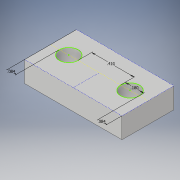
# Autodesk Inventor part: Rectangular Bottom Washer v1.2
Saved by Autodesk Inventor 2019 (Build 230136000, 136)
## iProperties
Created: 2020-01-11
Part Number: Rectangular Bottom Washer v1.2
Material: Generic
Document SubType Name: Modeling
Designer: Obscure_Decision
Density: 1 g/cm^3
Appearance: Default
Author: Obscure_Decision
Autodesk Inventor part; units mm, degrees
ref_plane "YZ Plane" through (0, 0, 0) normal (1, 0, 0) x (0, 1, 0)
ref_plane "XZ Plane" through (0, 0, 0) normal (0, 1, 0) x (-1, 0, 0)
ref_plane "XY Plane" through (0, 0, 0) normal (0, 0, 1) x (1, 0, 0)
sketch "Spacer 2D" plane through (0, 0, 0) normal (0, 1, 0) x (-1, 0, 0)
  line L0 (12.4883, 0) -> (12.4883, -12.7) construction
  line L1 (24.4009, -12.7) -> (0.5757, -12.7)
  line L2 (0.5757, -12.7) -> (0.5757, 0)
  line L3 (0.5757, 0) -> (24.4009, 0)
  line L4 (24.4009, 0) -> (24.4009, -12.7)
  line L5 (24.4009, -12.7) -> (0.5757, 0) construction
  line L6 (0.5757, -12.7) -> (24.4009, 0) construction
  point P0 (0, 0)
  point P1 (12.4883, -6.35)
  dimension "d17" = 23.8252
  dimension "d18" = 12.7
  constraints: 14 end point, 3 midpoint, 2 parallel, 1 horizontal, 1 perpendicular
  measures "d17" distance of L2.end L3.end
  measures "d18" distance of L3.end L1.start
extrude "Spacer Body" add sketch "Spacer 2D" along normal blind 5.08
sketch "Spacer Circles" plane through (0, 5.08, 0) normal (0, 1, 0) x (1, 0, 0)
  line L0 (-0.5757, 0) -> (-0.5757, 12.7) construction
  line L1 (-7.2813, 6.35) -> (-0.5757, 6.35) construction
  line L2 (-7.2813, 6.35) -> (-2.7093, 6.35) construction
  circle A0 centre (-4.9953, 6.35) radius 2.286
  line L3 (-17.6953, 6.35) -> (-7.2813, 6.35) construction
  line L4 (-17.6953, 6.35) -> (-24.4009, 6.35) construction
  line L5 (-24.4009, 12.7) -> (-24.4009, 0) construction
  line L6 (-0.5757, 0) -> (-24.4009, 0) construction
  line L7 (-24.4009, 0) -> (-24.4009, 12.7) construction
  line L8 (-24.4009, 12.7) -> (-0.5757, 12.7) construction
  line L9 (-0.5757, 12.7) -> (-0.5757, 0) construction
  line L10 (-12.4883, 6.35) -> (-12.4883, 0) construction
  line L11 (-24.4009, 0) -> (-0.5757, 0) construction
  circle A1 centre (-19.9813, 6.35) radius 2.286
  dimension "d25" = 4.572
  dimension "d26" = 10.414
  dimension "d31" = 2.1336
  dimension "d32" = 2.1336
  constraints: 18 end point, 5 midpoint, 2 horizontal, 2 parallel, 2 perpendicular, 1 centre point, 1 horizontal alignment, 1 point on line, 1 symmetric about line, 3 other
  measures "d25" distance of L1.start L2.end
  measures "d26" distance of L3.start L1.start
  measures "d31" distance from line of L2.end L0
  measures "d32" distance edge to line of A1 L5
extrude "Spacer Holes" cut sketch "Spacer Circles" against normal blind 10.16
body "Solid1"
